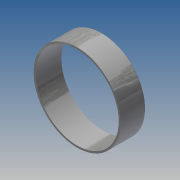
# Autodesk Inventor part: A1-19037-200-03 34in pipe
Saved by Autodesk Inventor 2017.3 (Build 213257000, 257)
## iProperties
Created: 2019-08-22
Part Number: A1-19037-200-03 34in pipe
Material: Steel, Mild
Document SubType Name: Modeling
Designer: GVD
Density: 7.85 g/cm^3
Appearance: Steel
Project: A1-19037--CNUL Albian CST laterals
Mass: 99260.1 g
Surface Area: 14361 cm^2
Volume: 12644.6 cm^3
Description: 34" x 3/4" WALL x 11 3/32" PIPE, API 5L X52 PSL-2
Constructed By: Graeme_Van_Dongen
Project Name: CST laterals
Author: GVD
Autodesk Inventor part; units mm, degrees
ref_plane "YZ Plane" through (0, 0, 0) normal (1, 0, 0) x (0, 1, 0)
ref_plane "XZ Plane" through (0, 0, 0) normal (0, 1, 0) x (-1, 0, 0)
sketch "Sketch1" plane through (0, 0, 0) normal (0, 0, 1) x (1, 0, 0)
  circle A0 centre (0, 0) radius 431.8
  circle A1 centre (0, 0) radius 412.75
  dimension "d0" = 863.6
  dimension "d1" = 825.5
  constraints: 2 centre point, 2 coincident
  measures "d0" diameter of A0
  measures "d1" diameter of A1
extrude "Extrusion1" add sketch "Sketch1" along normal blind 256.3812
chamfer "Chamfer1" distance 17.4625 angle 37.5 1 edges at (-431.8, 0, 0) measured on face at (-425.2038, 4.7488, 0)
ref_plane "Work Plane2" through (0, 0, 224.6312) normal (0, 0, 1) x (1, 0, 0)
ref_plane "Work Plane1" through (0, 0, 205.5812) normal (0, 0, 1) x (1, 0, 0)
split_face "Split1"
split_face "Split2"
chamfer "Chamfer2" distance 0.7937 angle 45 1 edges at (-412.75, 0, 256.3812)
body "Solid1"
